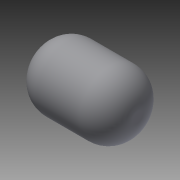
# Autodesk Inventor part: DMJ_Head
Saved by Autodesk Inventor 2015 SP1 (Build 190203100, 203)
## iProperties
Created: 2016-02-03
Part Number: DMJ_Head
Material: Generic
Document SubType Name: Modeling
Designer: guillemd
Density: 1 g/cm^3
Appearance: Default
Author: guillemd
Autodesk Inventor part; units mm, degrees
ref_plane "YZ Plane" through (0, 0, 0) normal (1, 0, 0) x (0, 1, 0)
ref_plane "XZ Plane" through (0, 0, 0) normal (0, 1, 0) x (-1, 0, 0)
ref_plane "XY Plane" through (0, 0, 0) normal (0, 0, 1) x (1, 0, 0)
sketch "Sketch1" plane through (0, 0, 0) normal (0, 1, 0) x (-1, 0, 0)
  line L0 (115.57, 0) -> (115.57, 12.7)
  line L1 (50.8, 77.47) -> (-50.8, 77.47)
  line L2 (-115.57, 12.7) -> (-115.57, 0)
  arc A0 (115.57, 12.7) -> (50.8, 77.47) centre (50.8, 12.7) ccw
  arc A1 (-50.8, 77.47) -> (-115.57, 12.7) centre (-50.8, 12.7) ccw
  line L3 (180.578, 0) -> (-180.578, 0) projected
  line L4 (115.57, 0) -> (-115.57, 0)
  point P0 (0, 0)
  point P1 (0, 77.47)
  dimension "d0" = 77.47
  dimension "d1" = 12.7
  dimension "d2" = 231.14
  constraints: 8 end point, 4 point on circle, 4 tangent, 2 centre point, 2 vertical, 1 collinear, 1 equal radius, 1 horizontal, 1 midpoint, 1 parallel, 1 point on line, 1 vertical alignment
  measures "d0" distance from line of L0.start L1
  measures "d1" distance of L0.start L0.end
  measures "d2" distance between parallel lines of L2 L0
revolve "Revolution1" add sketch "Sketch1" angle 360 about axis through (-10, 0, 0) along (1, 0, 0)
body "Solid1"
